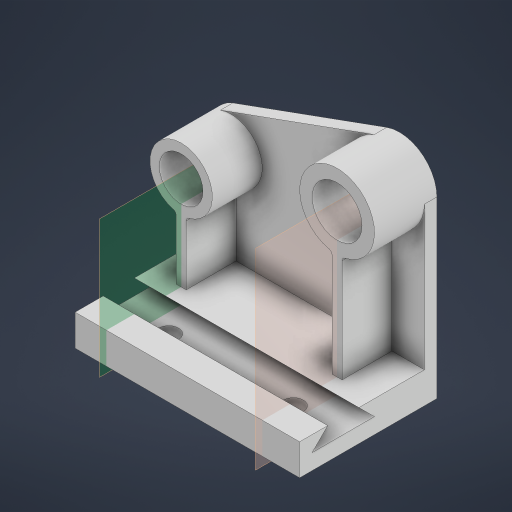
# Autodesk Inventor part: Część22
Saved by Autodesk Inventor 2023 (Build 270158000, 158)
## iProperties
Created: 2023-05-09
Part Number: Część22
Material: Ogólny
Document SubType Name: Modeling
Designer: Adam
Density: 1 g/cm^3
Appearance: Domyślna
Author: Adam
Autodesk Inventor part; units mm, degrees
ref_plane "YZ Plane" through (0, 0, 0) normal (1, 0, 0) x (0, 1, 0)
ref_plane "XZ Plane" through (0, 0, 0) normal (0, 1, 0) x (-1, 0, 0)
ref_plane "XY Plane" through (0, 0, 0) normal (0, 0, 1) x (1, 0, 0)
sketch "Szkic1" plane through (0, 0, 0) normal (0, 1, 0) x (-1, 0, 0)
  line L0 (0, 0) -> (-180, 0)
  line L1 (-180, 0) -> (-180, 110)
  line L2 (-180, 110) -> (0, 110)
  line L3 (0, 110) -> (0, 0)
  dimension "d0" = 180
  dimension "d1" = 110
  constraints: 8 end point, 2 parallel, 1 horizontal, 1 perpendicular
  measures "d0" distance of L1.end L2.end
  measures "d1" distance of L0.end L1.end
extrude "Wyciągnięcie proste1" add sketch "Szkic1" along normal blind 25
sketch "Szkic2" plane through (180, 0, 110) normal (1, 0, 0) x (0, 0, -1)
  line L0 (35, 25) -> (22.5, 25)
  line L1 (0, 25) -> (110, 25) projected
  line L2 (22.5, 25) -> (10, 12.5)
  line L3 (10, 12.5) -> (35, 12.5)
  line L4 (0, 0) -> (0, 25) projected
  line L5 (35, 25) -> (47.5, 25)
  line L6 (47.5, 25) -> (60, 12.5)
  line L7 (60, 12.5) -> (35, 12.5)
  point P0 (110, 0)
  point P1 (0, 12.5)
  dimension "d4" = 12.5
  dimension "d5" = 35
  dimension "d6" = 12.5
  dimension "d7" = 25
  dimension "d8" = 10
  constraints: 12 end point, 1 horizontal, 1 midpoint, 1 point on line
  measures "d4" distance of L0.start L0.end
  measures "d5" distance of L1.start L0.start
  measures "d6" distance between parallel lines of L3 L0
  measures "d7" distance of L3.end L2.end
  measures "d8" distance of point (0, 12.5) L2.end
extrude "Wyciągnięcie proste2" cut sketch "Szkic2" against normal through all
sketch "Szkic3" plane through (180, 12.5, 100) normal (0, 1, 0) x (1, 0, 0)
  point P0 (-180, 100)
sketch "Szkic4" plane through (180, 12.5, 100) normal (0, 1, 0) x (1, 0, 0)
  point P0 (-180, 100)
  point P1 (-140, 25)
  point P2 (-40, 25)
hole "Otwór1" at (140, 12.5, 75) at (40, 12.5, 75) direction (0, -1, 0) diameter 16 end through all
sketch "Szkic5" plane through (0, 0, 0) normal (0, 0, 1) x (1, 0, 0)
  circle A0 centre (150, 140) radius 30
  circle A1 centre (25, 100) radius 25
  line L0 (0, 25) -> (180, 25) projected
  line L1 (180, 25) -> (180, 140)
  line L2 (0, 25) -> (0, 12.5) projected
  line L3 (0, 25) -> (0, 100)
  line L4 (139.7748, 168.2037) -> (16.479, 123.503)
  point P0 (0, 0)
  dimension "d18" = 60
  dimension "d19" = 50
  dimension "d20" = 115
  dimension "d21" = 75
  constraints: 6 end point, 4 point on circle, 4 tangent, 2 centre point, 1 collinear, 1 vertical
  measures "d18" diameter of A0
  measures "d19" diameter of A1
  measures "d20" distance of L0.end L1.end
  measures "d21" distance of L0.start L3.end
extrude "Wyciągnięcie proste3" add sketch "Szkic5" along normal blind 10
sketch "Szkic6" plane through (0, 0, 10) normal (0, 0, 1) x (1, 0, 0)
  arc A0 (16.479, 123.503) -> (0, 100) centre (25, 100) ccw projected
  circle A1 centre (25, 100) radius 25
  arc A2 (180, 140) -> (139.7748, 168.2037) centre (150, 140) ccw projected
  circle A3 centre (150, 140) radius 30
  point P0 (0, 0)
  point P1 (0, 100)
  point P2 (16.479, 123.503)
  dimension "d41" = 50
  dimension "d42" = 60
  constraints: 2 centre point, 2 coincident
  measures "d41" diameter of A1
  measures "d42" diameter of A3
extrude "Wyciągnięcie proste4" add sketch "Szkic6" along normal blind 40
sketch "Szkic11" plane through (0, 0, 50) normal (0, 0, 1) x (1, 0, 0)
  point P0 (0, 0)
ref_plane "Płaszczyzna konstrukcyjna5" through (150, 0, 110) normal (1, 0, 0) x (0, 0, -1)
sketch "Szkic12" plane through (150, 0, 110) normal (1, 0, 0) x (0, 0, -1)
  line L0 (60, 125) -> (60, 75) projected
  line L1 (60, 75) -> (60, 25)
  line L2 (100, 25) -> (47.5, 25) projected
  point P0 (110, 0)
  constraints: 2 end point, 1 point on line, 1 vertical
extrude "Żebro3" add sketch "Szkic12" along normal mid plane 8 rib yes fills toward (60.05, 100) open curves L0 L1
ref_plane "Płaszczyzna konstrukcyjna6" through (25, 0, 0) normal (-1, 0, 0) x (0, 0, 1)
sketch "Szkic16" plane through (25, 0, 0) normal (-1, 0, 0) x (0, 0, 1)
  line L0 (50, 75) -> (50, 125) projected
  line L1 (50, 25) -> (50, 75)
  point P0 (0, 0)
  constraints: 2 end point, 1 collinear
extrude "Żebro4" add sketch "Szkic16" along normal mid plane 8 rib yes fills toward (49.95, 50) open curves L1 L0
fillet "Zaokrąglenie2" radius 3 4 edges at (21, 75.3221, 30) (29, 75.3221, 30) (154, 110.2679, 30) (146, 110.2679, 30)
sketch "Szkic17" plane through (0, 0, 50) normal (0, 0, 1) x (1, 0, 0)
  arc A0 (31.25, 75.7939) -> (16.479, 123.503) centre (25, 100) ccw projected
  point P0 (0, 0)
  constraints: 1 coincident
hole "Otwór2" at (25, 100, 50) direction (0, 0, -1) diameter 35 end through all
sketch "Szkic18" plane through (0, 0, 50) normal (0, 0, 1) x (1, 0, 0)
  arc A0 (156.3636, 110.6827) -> (143.6364, 110.6827) centre (150, 140) ccw projected
  point P0 (0, 0)
  constraints: 1 coincident
hole "Otwór3" at (150, 140, 50) direction (0, 0, -1) diameter 30 end through all counterbore diameter 40 counterbore depth 40
